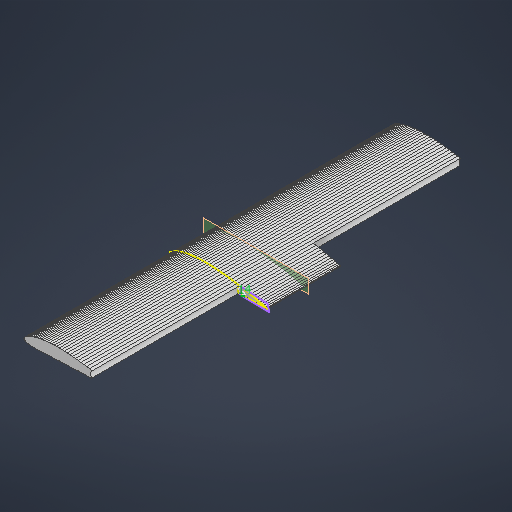
# Autodesk Inventor part: pokus 1
Saved by Autodesk Inventor 2026 (Build 300175050, 175E)
## iProperties
Created: 2026-01-16
Part Number: pokus 1
Material: Všeobecné
Document SubType Name: Modeling
Designer: marti
Density: 1 g/cm^3
Appearance: Výchozí
Author: marti
Autodesk Inventor part; units mm, degrees
ref_plane "YZ Plane" through (0, 0, 0) normal (1, 0, 0) x (0, 1, 0)
ref_plane "XZ Plane" through (0, 0, 0) normal (0, 1, 0) x (-1, 0, 0)
sketch "Náčrt3" plane through (0, 0, 0) normal (0, 0, 1) x (1, 0, 0)
  line L0 (0, 0) -> (0.1008, -0.6172)
  line L1 (0.1008, -0.6172) -> (0.4005, -1.1751)
  line L2 (0.4005, -1.1751) -> (0.8948, -1.675)
  line L3 (0.8948, -1.675) -> (1.5794, -2.1181)
  line L4 (1.5794, -2.1181) -> (2.45, -2.5059)
  line L5 (2.45, -2.5059) -> (3.502, -2.8399)
  line L6 (3.502, -2.8399) -> (4.7309, -3.1217)
  line L7 (4.7309, -3.1217) -> (6.1321, -3.3532)
  line L8 (6.1321, -3.3532) -> (7.7009, -3.5364)
  line L9 (7.7009, -3.5364) -> (9.4326, -3.6734)
  line L10 (9.4326, -3.6734) -> (11.3221, -3.7667)
  line L11 (11.3221, -3.7667) -> (13.3646, -3.8188)
  line L12 (13.3646, -3.8188) -> (15.5549, -3.8188)
  line L13 (15.5549, -3.8188) -> (17.8877, -3.8188)
  line L14 (17.8877, -3.8188) -> (20.3578, -3.7585)
  line L15 (20.3578, -3.7585) -> (22.9603, -3.695)
  line L16 (22.9603, -3.695) -> (25.688, -3.5719)
  line L17 (25.688, -3.5719) -> (28.5365, -3.4433)
  line L18 (28.5365, -3.4433) -> (31.5001, -3.3096)
  line L19 (31.5001, -3.3096) -> (34.5717, -3.1509)
  line L20 (34.5717, -3.1509) -> (37.7458, -2.9903)
  line L21 (37.7458, -2.9903) -> (41.0158, -2.8272)
  line L22 (41.0158, -2.8272) -> (44.3749, -2.6597)
  line L23 (44.3749, -2.6597) -> (47.817, -2.512)
  line L24 (47.817, -2.512) -> (51.3342, -2.369)
  line L25 (51.3342, -2.369) -> (54.9194, -2.2327)
  line L26 (54.9194, -2.2327) -> (58.5651, -2.0885)
  line L27 (58.5651, -2.0885) -> (62.2634, -1.9385)
  line L28 (62.2634, -1.9385) -> (66.0059, -1.7856)
  line L29 (66.0059, -1.7856) -> (69.7841, -1.632)
  line L30 (69.7841, -1.632) -> (73.5888, -1.4803)
  line L31 (73.5888, -1.4803) -> (77.4106, -1.3325)
  line L32 (77.4106, -1.3325) -> (85.0644, -1.0556)
  line L33 (85.0644, -1.0556) -> (88.8745, -0.9296)
  line L34 (88.8745, -0.9296) -> (92.6573, -0.8132)
  line L35 (92.6573, -0.8132) -> (96.3998, -0.7072)
  line L36 (96.3998, -0.7072) -> (100.0878, -0.612)
  line L37 (100.0878, -0.612) -> (103.7057, -0.5276)
  line L38 (103.7057, -0.5276) -> (107.2363, -0.4539)
  line L39 (107.2363, -0.4539) -> (110.6603, -0.3905)
  line L40 (110.6603, -0.3905) -> (113.9558, -0.3368)
  line L41 (113.9558, -0.3368) -> (117.0974, -0.2918)
  line L42 (117.0974, -0.2918) -> (120.055, -0.2549)
  line L43 (120.055, -0.2549) -> (122.7911, -0.2251)
  line L44 (122.7911, -0.2251) -> (125.2574, -0.2014)
  line L45 (125.2574, -0.2014) -> (127.3856, -0.1834)
  line L46 (127.3856, -0.1834) -> (129.0641, -0.1691)
  line L47 (129.0641, -0.1691) -> (129.9931, -0.1612)
  line L48 (129.9931, -0.1612) -> (129.9906, 0.1321)
  line L49 (129.9906, 0.1321) -> (129.0576, 0.3875)
  line L50 (129.0576, 0.3875) -> (127.3795, 0.839)
  line L51 (127.3795, 0.839) -> (125.2516, 1.3993)
  line L52 (125.2516, 1.3993) -> (122.7858, 2.032)
  line L53 (122.7858, 2.032) -> (120.0501, 2.7132)
  line L54 (120.0501, 2.7132) -> (117.0931, 3.4254)
  line L55 (117.0931, 3.4254) -> (113.952, 4.1548)
  line L56 (113.952, 4.1548) -> (110.657, 4.8904)
  line L57 (110.657, 4.8904) -> (107.2335, 5.6228)
  line L58 (107.2335, 5.6228) -> (103.7034, 6.3444)
  line L59 (103.7034, 6.3444) -> (100.086, 7.0485)
  line L60 (100.086, 7.0485) -> (96.3985, 7.7294)
  line L61 (96.3985, 7.7294) -> (92.6565, 8.3822)
  line L62 (92.6565, 8.3822) -> (88.8741, 9.0026)
  line L63 (88.8741, 9.0026) -> (85.0644, 9.5868)
  line L64 (85.0644, 9.5868) -> (81.2394, 10.1289)
  line L65 (81.2394, 10.1289) -> (77.4106, 10.6287)
  line L66 (77.4106, 10.6287) -> (73.5888, 11.0836)
  line L67 (73.5888, 11.0836) -> (69.7841, 11.4914)
  line L68 (69.7841, 11.4914) -> (66.0059, 11.8502)
  line L69 (66.0059, 11.8502) -> (62.2634, 12.1585)
  line L70 (62.2634, 12.1585) -> (58.5651, 12.4148)
  line L71 (58.5651, 12.4148) -> (54.9194, 12.6181)
  line L72 (54.9194, 12.6181) -> (51.3342, 12.7673)
  line L73 (51.3342, 12.7673) -> (47.817, 12.8447)
  line L74 (47.817, 12.8447) -> (44.3752, 12.8426)
  line L75 (44.3752, 12.8426) -> (41.0158, 12.7632)
  line L76 (41.0158, 12.7632) -> (37.7458, 12.6088)
  line L77 (37.7458, 12.6088) -> (34.5717, 12.3826)
  line L78 (34.5717, 12.3826) -> (31.4999, 12.088)
  line L79 (31.4999, 12.088) -> (28.5366, 11.7287)
  line L80 (28.5366, 11.7287) -> (25.688, 11.3091)
  line L81 (25.688, 11.3091) -> (22.9598, 10.8338)
  line L82 (22.9598, 10.8338) -> (20.3578, 10.3077)
  line L83 (20.3578, 10.3077) -> (17.8877, 9.7359)
  line L84 (17.8877, 9.7359) -> (15.5548, 9.1241)
  line L85 (15.5548, 9.1241) -> (13.3646, 8.4777)
  line L86 (13.3646, 8.4777) -> (11.3221, 7.8025)
  line L87 (11.3221, 7.8025) -> (9.4326, 7.1042)
  line L88 (9.4326, 7.1042) -> (7.7009, 6.3887)
  line L89 (7.7009, 6.3887) -> (6.1321, 5.6614)
  line L90 (6.1321, 5.6614) -> (4.7309, 4.928)
  line L91 (4.7309, 4.928) -> (3.502, 4.1935)
  line L92 (3.502, 4.1935) -> (2.45, 3.4628)
  line L93 (2.45, 3.4628) -> (1.5794, 2.7403)
  line L94 (1.5794, 2.7403) -> (0.8948, 2.0298)
  line L95 (0.8948, 2.0298) -> (0.4005, 1.3347)
  line L96 (0.4005, 1.3347) -> (0.1008, 0.6574)
  line L97 (0.1008, 0.6574) -> (0, 0)
  point P0 (81.2394, -1.1904)
  constraints: 196 end point, 7 collinear, 2 perpendicular, 1 horizontal, 1 parallel
extrude "Vysunutí1" add sketch "Náčrt3" along normal mid plane 500
sketch "Náčrt4" plane through (0, 0, 250) normal (0, 0, 1) x (1, 0, 0)
  line L0 (92.6573, -0.8132) -> (88.8745, -0.9296) projected
  line L1 (92.6565, 8.3822) -> (96.3985, 7.7294) projected
  arc A0 (92.6565, 8.3822) -> (91.7048, -0.8425) centre (98.1463, 3.1544) ccw
  line L2 (91.7048, -0.8425) -> (107.6986, -0.3505)
  line L3 (129.9931, -0.1612) -> (125.2574, -0.2014) projected
  line L4 (107.6986, -0.3505) -> (129.9931, -0.1612)
  line L5 (129.9906, 0.1321) -> (129.0576, 0.3875) projected
  line L6 (129.9931, -0.1612) -> (129.9906, 0.1321)
  line L7 (129.9906, 0.1321) -> (93.9107, 9.4415)
  line L8 (93.9107, 9.4415) -> (92.6565, 8.3822)
  line L9 (91.7048, -0.8425) -> (93.0009, -2.4127)
  line L10 (93.0009, -2.4127) -> (129.9931, -0.1612)
  line L11 (129.9931, -0.1612) -> (130.1118, -0.1429)
  line L12 (130.1118, -0.1429) -> (130.1094, 0.1331)
  line L13 (130.1094, 0.1331) -> (129.9906, 0.1321)
  line L14 (130.1094, 0.1331) -> (128.1613, 1.4193)
  line L15 (128.1613, 1.4193) -> (113.3536, 4.4248)
  point P0 (0, 0)
  constraints: 24 end point, 4 point on circle, 4 point on line, 2 perpendicular, 1 centre point
extrude "Vysunutí2" cut sketch "Náčrt4" against normal blind 200
mirror "Zrcadlit1" about plane through (0, 0, 0) normal (0, 0, 1) of "Vysunutí2"
sketch "Náčrt6" plane through (0, 0, 50) normal (0, 0, 1) x (1, 0, 0)
  arc A0 (92.6565, 8.3822) -> (91.7048, -0.8425) centre (98.1463, 3.1544) ccw projected
  line L0 (92.6565, 8.3822) -> (96.3985, 7.7294) projected
  arc A1 (92.6565, 8.3822) -> (91.7048, -0.8425) centre (98.1463, 3.1544) ccw projected
  line L1 (92.6573, -0.8132) -> (91.7048, -0.8425) projected
  line L2 (96.3998, -0.7072) -> (92.6573, -0.8132) projected
  line L3 (100.0878, -0.612) -> (96.3998, -0.7072) projected
  line L4 (103.7057, -0.5276) -> (100.0878, -0.612) projected
  line L5 (107.2363, -0.4539) -> (103.7057, -0.5276) projected
  line L6 (110.6603, -0.3905) -> (107.2363, -0.4539) projected
  line L7 (113.9558, -0.3368) -> (110.6603, -0.3905) projected
  line L8 (117.0974, -0.2918) -> (113.9558, -0.3368) projected
  line L9 (120.055, -0.2549) -> (117.0974, -0.2918) projected
  line L10 (122.7911, -0.2251) -> (120.055, -0.2549) projected
  line L11 (125.2574, -0.2014) -> (122.7911, -0.2251) projected
  line L12 (129.9931, -0.1612) -> (125.2574, -0.2014) projected
  line L13 (129.9906, 0.1321) -> (129.9931, -0.1612) projected
  line L14 (129.0576, 0.3875) -> (129.9906, 0.1321) projected
  line L15 (127.3795, 0.839) -> (129.0576, 0.3875) projected
  line L16 (125.2516, 1.3993) -> (127.3795, 0.839) projected
  line L17 (122.7858, 2.032) -> (125.2516, 1.3993) projected
  line L18 (120.0501, 2.7132) -> (122.7858, 2.032) projected
  line L19 (117.0931, 3.4254) -> (120.0501, 2.7132) projected
  line L20 (113.952, 4.1548) -> (117.0931, 3.4254) projected
  line L21 (110.657, 4.8904) -> (113.952, 4.1548) projected
  line L22 (107.2335, 5.6228) -> (110.657, 4.8904) projected
  line L23 (103.7034, 6.3444) -> (107.2335, 5.6228) projected
  line L24 (100.086, 7.0485) -> (103.7034, 6.3444) projected
  line L25 (96.3985, 7.7294) -> (100.086, 7.0485) projected
  arc A2 (92.6565, 8.3822) -> (91.7048, -0.8425) centre (98.1463, 3.1544) ccw projected
  line L26 (92.6565, 8.3822) -> (88.8741, 9.0026) projected
  line L27 (88.8741, 9.0026) -> (85.0644, 9.5868) projected
  line L28 (85.0644, 9.5868) -> (81.2394, 10.1289) projected
  line L29 (81.2394, 10.1289) -> (77.4106, 10.6287) projected
  line L30 (77.4106, 10.6287) -> (73.5888, 11.0836) projected
  line L31 (73.5888, 11.0836) -> (69.7841, 11.4914) projected
  line L32 (69.7841, 11.4914) -> (66.0059, 11.8502) projected
  line L33 (66.0059, 11.8502) -> (62.2634, 12.1585) projected
  line L34 (62.2634, 12.1585) -> (58.5651, 12.4148) projected
  line L35 (58.5651, 12.4148) -> (54.9194, 12.6181) projected
  line L36 (54.9194, 12.6181) -> (51.3342, 12.7673) projected
  line L37 (51.3342, 12.7673) -> (47.817, 12.8447) projected
  line L38 (47.817, 12.8447) -> (44.3752, 12.8426) projected
  line L39 (44.3752, 12.8426) -> (41.0158, 12.7632) projected
  line L40 (41.0158, 12.7632) -> (37.7458, 12.6088) projected
  line L41 (37.7458, 12.6088) -> (34.5717, 12.3826) projected
  line L42 (34.5717, 12.3826) -> (31.4999, 12.088) projected
  line L43 (31.4999, 12.088) -> (28.5366, 11.7287) projected
  line L44 (28.5366, 11.7287) -> (25.688, 11.3091) projected
  line L45 (25.688, 11.3091) -> (22.9598, 10.8338) projected
  line L46 (22.9598, 10.8338) -> (20.3578, 10.3077) projected
  line L47 (20.3578, 10.3077) -> (17.8877, 9.7359) projected
  line L48 (17.8877, 9.7359) -> (15.5548, 9.1241) projected
  line L49 (15.5548, 9.1241) -> (13.3646, 8.4777) projected
  line L50 (13.3646, 8.4777) -> (11.3221, 7.8025) projected
  line L51 (11.3221, 7.8025) -> (9.4326, 7.1042) projected
  line L52 (9.4326, 7.1042) -> (7.7009, 6.3887) projected
  line L53 (7.7009, 6.3887) -> (6.1321, 5.6614) projected
  line L54 (6.1321, 5.6614) -> (4.7309, 4.928) projected
  line L55 (4.7309, 4.928) -> (3.502, 4.1935) projected
  line L56 (3.502, 4.1935) -> (2.45, 3.4628) projected
  line L57 (2.45, 3.4628) -> (1.5794, 2.7403) projected
  line L58 (1.5794, 2.7403) -> (0.8948, 2.0298) projected
  line L59 (0.8948, 2.0298) -> (0.4005, 1.3347) projected
  line L60 (0.4005, 1.3347) -> (0.1008, 0.6574) projected
  line L61 (0.1008, 0.6574) -> (0, 0) projected
  line L62 (0, 0) -> (0.1008, -0.6172) projected
  line L63 (0.1008, -0.6172) -> (0.4005, -1.1751) projected
  line L64 (0.4005, -1.1751) -> (0.8948, -1.675) projected
  line L65 (0.8948, -1.675) -> (1.5794, -2.1181) projected
  line L66 (1.5794, -2.1181) -> (2.45, -2.5059) projected
  line L67 (2.45, -2.5059) -> (3.502, -2.8399) projected
  line L68 (3.502, -2.8399) -> (4.7309, -3.1217) projected
  line L69 (4.7309, -3.1217) -> (6.1321, -3.3532) projected
  line L70 (6.1321, -3.3532) -> (7.7009, -3.5364) projected
  line L71 (7.7009, -3.5364) -> (9.4326, -3.6734) projected
  line L72 (9.4326, -3.6734) -> (11.3221, -3.7667) projected
  line L73 (11.3221, -3.7667) -> (13.3646, -3.8188) projected
  line L74 (13.3646, -3.8188) -> (17.8877, -3.8188) projected
  line L75 (17.8877, -3.8188) -> (22.9603, -3.695) projected
  line L76 (22.9603, -3.695) -> (31.5001, -3.3096) projected
  line L77 (31.5001, -3.3096) -> (34.5717, -3.1509) projected
  line L78 (34.5717, -3.1509) -> (37.7458, -2.9903) projected
  line L79 (37.7458, -2.9903) -> (44.3749, -2.6597) projected
  line L80 (44.3749, -2.6597) -> (47.817, -2.512) projected
  line L81 (47.817, -2.512) -> (51.3342, -2.369) projected
  line L82 (51.3342, -2.369) -> (54.9194, -2.2327) projected
  line L83 (54.9194, -2.2327) -> (58.5651, -2.0885) projected
  line L84 (58.5651, -2.0885) -> (62.2634, -1.9385) projected
  line L85 (62.2634, -1.9385) -> (66.0059, -1.7856) projected
  line L86 (66.0059, -1.7856) -> (69.7841, -1.632) projected
  line L87 (69.7841, -1.632) -> (73.5888, -1.4803) projected
  line L88 (73.5888, -1.4803) -> (77.4106, -1.3325) projected
  line L89 (77.4106, -1.3325) -> (85.0644, -1.0556) projected
  line L90 (85.0644, -1.0556) -> (88.8745, -0.9296) projected
  line L91 (88.8745, -0.9296) -> (91.7048, -0.8425) projected
  arc A3 (93.3574, 8.2599) -> (92.3851, -0.8216) centre (98.1463, 3.1544) ccw
  line L92 (93.3574, 8.2599) -> (130.682, 6.3444)
  line L93 (130.682, 6.3444) -> (133.047, -2.512)
  line L94 (133.047, -2.512) -> (94.9361, -1.9385)
  line L95 (94.9361, -1.9385) -> (92.3851, -0.8216)
  point P0 (92.6565, 8.3822)
  point P1 (91.7048, -0.8425)
  dimension "d7" = 14
  constraints: 8 end point, 2 point on circle, 2 point on line, 1 centre point, 1 coincident
  measures "d7" diameter of A3
ref_plane "Pracovní rovina1" through (0, 0, 0) normal (0, 0, 1) x (1, 0, 0)
